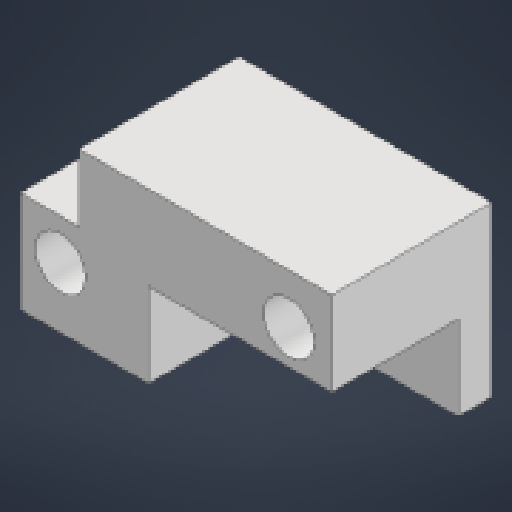
# Autodesk Inventor part: 固定传动
Saved by Autodesk Inventor 2025 (Build 290162000, 162)
## iProperties
Created: 2025-12-09
Part Number: 固定传动
Material: 常规
Document SubType Name: Modeling
Designer: XH
Density: 1 g/cm^3
Appearance: 默认
Author: XH
Autodesk Inventor part; units mm, degrees
ref_plane "YZ Plane" through (0, 0, 0) normal (1, 0, 0) x (0, 1, 0)
ref_plane "XZ Plane" through (0, 0, 0) normal (0, 1, 0) x (-1, 0, 0)
ref_plane "XY Plane" through (0, 0, 0) normal (0, 0, 1) x (1, 0, 0)
sketch "草图1" plane through (0, 0, 0) normal (0, 0, 1) x (1, 0, 0)
  line L0 (-22.2679, -12.5636) -> (-1.2679, -12.5636) projected
  line L1 (-24.2679, 7.4364) -> (5.7321, 7.4364)
  line L2 (5.7321, 7.4364) -> (5.7321, -12.5636)
  line L3 (5.7321, -12.5636) -> (-24.2679, -12.5636)
  line L4 (-24.2679, -12.5636) -> (-24.2679, 7.4364)
  point P0 (-22.2679, -12.5636)
  point P1 (-1.2679, -12.5636)
  dimension "d4" = 30
  dimension "d5" = 20
  constraints: 8 end point, 2 parallel, 1 collinear, 1 horizontal, 1 perpendicular
  measures "d4" distance of L1.start L1.end
  measures "d5" distance of L1.end L2.end
extrude "拉伸1" add sketch "草图1" along normal blind 19
sketch "草图2" plane through (0, 0, 0) normal (0, 0, -1) x (-1, 0, 0)
  line L0 (24.2679, 7.4364) -> (24.2679, -12.5636) projected
  line L1 (24.2679, -12.5636) -> (31.2679, -12.5636)
  line L2 (31.2679, -12.5636) -> (31.2679, -0.5636)
  line L3 (31.2679, -0.5636) -> (24.2679, -0.5636)
  line L4 (24.2679, -0.5636) -> (24.2679, -12.5636)
  point P0 (0, 0)
  dimension "d6" = 7
  dimension "d7" = 12
  constraints: 8 end point, 2 parallel, 1 horizontal, 1 perpendicular
  measures "d6" distance of L2.end L3.end
  measures "d7" distance of L1.end L2.end
extrude "拉伸2" add sketch "草图2" against normal up to surface (19 mm away)
sketch "草图3" plane through (0, 0, 0) normal (0, 0, -1) x (-1, 0, 0)
  circle A0 centre (-0.6256, 1.5535) radius 3
  circle A1 centre (26.4728, -5.3671) radius 3
  point P0 (0, 0)
  dimension "d10" = 6
  dimension "d11" = 6
  constraints: 2 centre point
  measures "d10" diameter of A0
  measures "d11" diameter of A1
extrude "拉伸3" cut sketch "草图3" against normal blind 40
sketch "草图4" plane through (5.7321, -12.5636, 0) normal (1, 0, 0) x (0, 0, -1)
  line L0 (-19, 0) -> (-4, 0)
  line L1 (-4, 0) -> (-4, 10)
  line L2 (-4, 10) -> (-19, 10)
  line L3 (-19, 10) -> (-19, 0)
  point P0 (0, 12.5636)
  dimension "d14" = 10
  dimension "d15" = 15
  constraints: 8 end point, 2 parallel, 1 horizontal, 1 perpendicular
  measures "d14" distance of L2.end L0.start
  measures "d15" distance of L1.end L2.end
extrude "拉伸4" cut sketch "草图4" against normal blind 21.75
chamfer "倒角1" distance 4 angle 45 1 edges at (-24.2679, -0.5636, 9.5)
